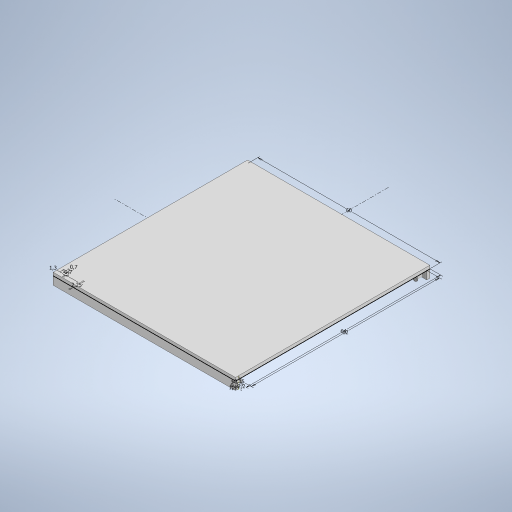
# Autodesk Inventor part: coperchio contieni SD
Saved by Autodesk Inventor 2023 (Build 270158000, 158)
## iProperties
Created: 2023-07-26
Part Number: coperchio contieni SD
Material: Generico
Document SubType Name: Modeling
Designer: Admin
Density: 1 g/cm^3
Appearance: Default
Author: Admin
Autodesk Inventor part; units mm, degrees
ref_plane "YZ Plane" through (0, 0, 0) normal (1, 0, 0) x (0, 1, 0)
ref_plane "XZ Plane" through (0, 0, 0) normal (0, 1, 0) x (-1, 0, 0)
ref_plane "XY Plane" through (0, 0, 0) normal (0, 0, 1) x (1, 0, 0)
sketch "Schizzo1" plane through (0, 0, 0) normal (0, 1, 0) x (-1, 0, 0)
  line L0 (30, 32) -> (-30, 32)
  line L1 (-30, 32) -> (-30, -32)
  line L2 (-30, -32) -> (30, -32)
  line L3 (30, -32) -> (30, 32)
  line L4 (0, 0) -> (41.9471, 0) construction
  line L5 (0, 0) -> (0, -48.4274) construction
  line L6 (28.8, 32) -> (28.8, 29.75) construction
  line L7 (28.8, 29.75) -> (30, 29.75) construction
  line L8 (28.8, 29.75) -> (28.1, 29.75) construction
  circle A0 centre (28.1, 29.75) radius 0.35
  line L9 (28.8, -32) -> (28.8, -29.75) construction
  line L10 (28.8, -29.75) -> (30, -29.75) construction
  line L11 (28.8, -29.75) -> (28.1, -29.75) construction
  circle A1 centre (28.1, -29.75) radius 0.7
  circle A2 centre (28.1, -29.75) radius 0.35
  circle A3 centre (28.1, 29.75) radius 0.65
  line L12 (30, 31) -> (-30, 31)
  line L13 (-30, 31) -> (-30, -31)
  line L14 (-30, -31) -> (30, -31)
  line L15 (30, -31) -> (30, 31)
  dimension "d0" = 60
  dimension "d1" = 64
  dimension "d2" = 2.25
  dimension "d3" = 1.2
  dimension "d4" = 0.7
  dimension "d5" = 0.7
  dimension "d8" = 1.3
  dimension "d9" = 62
  constraints: 32 end point, 5 symmetric about line, 4 horizontal, 4 parallel, 4 point on line, 3 centre point, 3 coincident, 3 perpendicular, 2 vertical, 1 horizontal alignment, 6 other
  measures "d0" distance of L2.end L1.end
  measures "d1" distance of L1.end L0.end
  measures "d2" distance of L6.start L6.end
  measures "d3" distance of L6.end L7.end
  measures "d4" distance of L8.start L8.end
  measures "d5" diameter of A0
  measures "d8" diameter of A3
  measures "d9" distance of L13.end L12.end
extrude "Estrusione1" add sketch "Schizzo1" along normal blind 1 contours L3 L12 L1 L0 | L3 L14 L1 L12 | L3 L2 L1 L14 | A0 | A1 | A2 | A3
extrude "Estrusione2" add sketch "Schizzo1" against normal blind 2.7 contours L3 L12 L1 L0 | L3 L2 L1 L14
sketch "Schizzo2" plane through (30, 0, 31) normal (0, 0, -1) x (-1, 0, 0)
  line L0 (0, -2.7) -> (60, -2.7) projected
  line L1 (0, -2.7) -> (0, 1) construction
  line L2 (0, -0.5) -> (6.4394, -0.5) construction
  line L3 (0, -0.5) -> (0, -0.65) construction
  line L4 (0, -0.65) -> (0, -2.15) construction
  line L5 (0, -2.15) -> (1, -2.15) construction
  line L6 (1, -2.15) -> (1.7, -2.15) construction
  circle A0 centre (1.7, -2.15) radius 0.7
  circle A1 centre (1.7, -2.15) radius 0.4
  line L7 (0, -0.5) -> (0, 0) construction
  point P0 (30, 0)
  dimension "d14" = 2.2
  dimension "d15" = 0.15
  dimension "d16" = 1.5
  dimension "d17" = 1
  dimension "d18" = 0.7
  dimension "d19" = 1.4
  dimension "d20" = 0.8
  constraints: 12 end point, 5 point on line, 2 centre point, 2 coincident, 2 horizontal
  measures "d14" distance of L0.start L2.start
  measures "d15" distance of L2.start L3.end
  measures "d16" distance of L3.end L4.end
  measures "d17" distance of L4.end L5.end
  measures "d18" distance of L5.end L6.end
  measures "d19" diameter of A0
  measures "d20" diameter of A1
extrude "Estrusione3" add sketch "Schizzo2" along normal blind 2.2 contours A0 L0 | L0 A0 | A1
extrude "Estrusione4" cut sketch "Schizzo2" along normal blind 1.9
sketch "Schizzo3" plane through (-30, 0, -31) normal (0, 0, 1) x (1, 0, 0)
  line L0 (60, -2.7) -> (60, 1) projected
  line L1 (0, -2.7) -> (60, -2.7) projected
  line L2 (60, 0) -> (60, -0.65) construction
  line L3 (60, -0.65) -> (60, -2.15) construction
  line L4 (60, -2.15) -> (59, -2.15) construction
  line L5 (59, -2.15) -> (58.3, -2.15) construction
  circle A0 centre (58.3, -2.15) radius 0.7
  circle A1 centre (58.3, -2.15) radius 0.4
  line L6 (0, 0) -> (60, 0) projected
  point P0 (30, 0)
  dimension "d26" = 0.65
  dimension "d27" = 1.5
  dimension "d28" = 1
  dimension "d29" = 0.7
  dimension "d30" = 1.4
  dimension "d31" = 0.8
  constraints: 8 end point, 5 point on line, 2 centre point, 2 coincident, 1 parallel, 1 perpendicular
  measures "d26" distance of L2.start L2.end
  measures "d27" distance of L2.end L3.end
  measures "d28" distance of L3.end L4.end
  measures "d29" distance of L4.end L5.end
  measures "d30" diameter of A0
  measures "d31" diameter of A1
extrude "Estrusione5" add sketch "Schizzo3" along normal blind 2.2 contours A0 L1 | L1 A0 | A1
extrude "Estrusione6" cut sketch "Schizzo3" along normal blind 1.9
